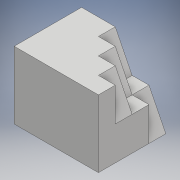
# Autodesk Inventor part: 23
Saved by Autodesk Inventor 2017 (Build 210142000, 142)
## iProperties
Part Number: 23
Material: 一般
Document SubType Name: Modeling
Designer: Brian
Density: 1 g/cm^3
Appearance: 預設
Author: Brian
Autodesk Inventor part; units mm, degrees
ref_plane "YZ Plane" through (0, 0, 0) normal (1, 0, 0) x (0, 1, 0)
ref_plane "XZ Plane" through (0, 0, 0) normal (0, 1, 0) x (-1, 0, 0)
ref_plane "XY Plane" through (0, 0, 0) normal (0, 0, 1) x (1, 0, 0)
sketch "草圖1" plane through (0, 0, 0) normal (0, 1, 0) x (-1, 0, 0)
  line L0 (0, 0) -> (-50, 0)
  line L1 (-50, 0) -> (-50, -40)
  line L2 (-50, -40) -> (0, -40)
  line L3 (0, -40) -> (0, 0)
  dimension "d0" = 40
  dimension "d1" = 50
  constraints: 8 end point, 2 parallel, 1 horizontal, 1 perpendicular
  measures "d0" distance of L2.end L0.start
  measures "d1" distance of L1.end L2.end
extrude "擠出1" add sketch "草圖1" along normal blind 40
sketch "草圖2" plane through (0, 40, 0) normal (0, 1, 0) x (1, 0, 0)
  line L0 (50, 0) -> (50, 40) projected
  line L1 (50, 40) -> (40, 20)
  line L2 (40, 20) -> (30, 20)
  line L3 (30, 20) -> (20, 0)
  line L4 (0, 0) -> (50, 0) projected
  dimension "d4" = 20
  dimension "d5" = 10
  dimension "d6" = 10
  dimension "d7" = 10
  constraints: 6 end point, 1 perpendicular, 1 point on line
  measures "d4" vertical distance of L0.end L1.end
  measures "d5" distance of L1.end L2.end
  measures "d6" horizontal distance of L2.end L3.end
  measures "d7" horizontal distance of L0.end L1.end
extrude "擠出2" cut sketch "草圖2" against normal blind 10
sketch "草圖3" plane through (0, 30, 0) normal (0, 1, 0) x (1, 0, 0)
  line L0 (30, 20) -> (40, 20) projected
  line L1 (40, 20) -> (30, 0)
  line L2 (50, 0) -> (20, 0) projected
  line L3 (40, 20) -> (50, 20)
  line L4 (50, 40) -> (50, 0) projected
  line L5 (50, 20) -> (50, 0)
  point P0 (0, 0)
  dimension "d10" = 10
  constraints: 6 end point, 1 midpoint, 1 point on line, 1 vertical
  measures "d10" horizontal distance of L0.end L1.end
extrude "擠出3" cut sketch "草圖3" against normal blind 10
sketch "草圖4" plane through (0, 20, 0) normal (0, 1, 0) x (1, 0, 0)
  line L0 (50, 20) -> (50, 0) projected
  line L1 (50, 20) -> (40, 0)
  line L2 (50, 0) -> (30, 0) projected
  point P0 (0, 0)
  dimension "d13" = 10
  constraints: 2 end point, 1 midpoint
  measures "d13" horizontal distance of L0.start L1.end
extrude "擠出4" cut sketch "草圖4" against normal blind 10
